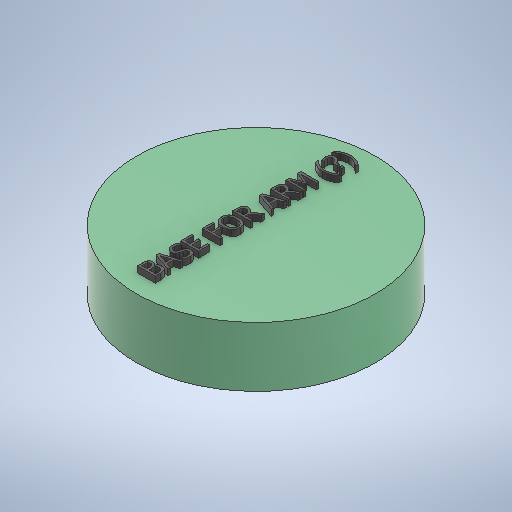
# Autodesk Inventor part: Base Mockup
Saved by Autodesk Inventor 2025.2 (Build 292293000, 293)
## iProperties
Created: 2025-01-24
Part Number: Base Mockup
Material: Generic
Document SubType Name: Modeling
Designer: Matt Tidd
Density: 1 g/cm^3
Appearance: Default
Author: Matt Tidd
Autodesk Inventor part; units mm, degrees
ref_plane "YZ Plane" through (0, 0, 0) normal (1, 0, 0) x (0, 1, 0)
ref_plane "XZ Plane" through (0, 0, 0) normal (0, 1, 0) x (-1, 0, 0)
ref_plane "XY Plane" through (0, 0, 0) normal (0, 0, 1) x (1, 0, 0)
sketch "Sketch1" plane through (0, 0, 0) normal (0, 1, 0) x (-1, 0, 0)
  circle A0 centre (0, 0) radius 50
  dimension "d0" = 100
  constraints: 1 centre point, 1 coincident
  measures "d0" diameter of A0
extrude "Extrusion1" add sketch "Sketch1" along normal blind 25
sketch "Sketch2" plane through (0, 25, 0) normal (0, 1, 0) x (1, 0, 0)
  line L0 (0, -50) -> (0, 50) construction
  circle A0 centre (0, 0) radius 50 projected
  spline S0 degree 2 poles (-2.3035, -37.0837) (-1.7443, -37.0837) (-0.8874, -37.5091) (-0.6078, -37.8616) knots 0 0 0 1 2 2 2
  spline S1 degree 2 poles (-0.6078, -37.8616) (-0.2796, -38.2871) (0, -39.2534) (0, -40.0192) knots 0 0 0 1 2 2 2
  line L1 (0, -40.0192) -> (0, -42.1708)
  line L2 (0, -42.1708) -> (-7.5, -42.1708)
  line L3 (-7.5, -42.1708) -> (-7.5, -40.1833)
  spline S2 degree 2 poles (-7.5, -40.1833) (-7.5, -39.3811) (-7.3967, -38.5788) (-7.1961, -38.2141) knots 0 0 0 1 2 2 2
  spline S3 degree 2 poles (-7.1961, -38.2141) (-6.9834, -37.8069) (-6.2844, -37.4362) (-5.8104, -37.4362) knots 0 0 0 1 2 2 2
  spline S4 degree 2 poles (-5.8104, -37.4362) (-5.2816, -37.4362) (-4.4429, -37.9953) (-4.2058, -38.4876) knots 0 0 0 1 2 2 2
  line L4 (-4.2058, -38.4876) -> (-4.1694, -38.4876)
  spline S5 degree 2 poles (-4.1694, -38.4876) (-3.987, -37.8191) (-3.0207, -37.0837) (-2.3035, -37.0837) knots 0 0 0 1 2 2 2
  spline S6 degree 2 poles (-2.2609, -38.123) (-2.6864, -38.123) (-3.2334, -38.3661) (-3.4279, -38.7308) knots 0 0 0 1 2 2 2
  spline S7 degree 2 poles (-3.4279, -38.7308) (-3.5494, -38.9678) (-3.6224, -39.5269) (-3.6224, -40.0436) knots 0 0 0 1 2 2 2
  line L5 (-3.6224, -40.0436) -> (-3.6224, -41.174)
  line L6 (-3.6224, -41.174) -> (-0.8509, -41.174)
  line L7 (-0.8509, -41.174) -> (-0.8509, -40.3657)
  spline S8 degree 2 poles (-0.8509, -40.3657) (-0.8509, -39.7093) (-0.9724, -38.9556) (-1.1669, -38.6639) knots 0 0 0 1 2 2 2
  spline S9 degree 2 poles (-1.1669, -38.6639) (-1.3675, -38.3843) (-1.8659, -38.123) (-2.2609, -38.123) knots 0 0 0 1 2 2 2
  spline S10 degree 2 poles (-5.6706, -38.4755) (-5.938, -38.4755) (-6.3391, -38.6578) (-6.4546, -38.8584) knots 0 0 0 1 2 2 2
  spline S11 degree 2 poles (-6.4546, -38.8584) (-6.5883, -39.1015) (-6.6491, -39.691) (-6.6491, -40.2198) knots 0 0 0 1 2 2 2
  line L8 (-6.6491, -40.2198) -> (-6.6491, -41.174)
  line L9 (-6.6491, -41.174) -> (-4.455, -41.174)
  line L10 (-4.455, -41.174) -> (-4.455, -40.0436)
  spline S12 degree 2 poles (-4.455, -40.0436) (-4.455, -39.5756) (-4.5523, -39.1319) (-4.7042, -38.8949) knots 0 0 0 1 2 2 2
  spline S13 degree 2 poles (-4.7042, -38.8949) (-4.8501, -38.6639) (-5.3181, -38.4755) (-5.6706, -38.4755) knots 0 0 0 1 2 2 2
  line L11 (0, -36.9013) -> (-7.5, -34.373)
  line L12 (-7.5, -34.373) -> (-7.5, -33.1453)
  line L13 (-7.5, -33.1453) -> (0, -30.6169)
  line L14 (0, -30.6169) -> (0, -31.6684)
  line L15 (0, -31.6684) -> (-2.0968, -32.3491)
  line L16 (-2.0968, -32.3491) -> (-2.0968, -35.2117)
  line L17 (-2.0968, -35.2117) -> (0, -35.8924)
  line L18 (0, -35.8924) -> (0, -36.9013)
  line L19 (-2.9477, -32.6226) -> (-6.4789, -33.7834)
  line L20 (-6.4789, -33.7834) -> (-2.9477, -34.9382)
  line L21 (-2.9477, -34.9382) -> (-2.9477, -32.6226)
  spline S14 degree 2 poles (0.1337, -27.7178) (0.1337, -28.5322) (-0.2066, -29.6748) (-0.4498, -30.1793) knots 0 0 0 1 2 2 2
  line L22 (-0.4498, -30.1793) -> (-1.7018, -30.1793)
  line L23 (-1.7018, -30.1793) -> (-1.7018, -30.1064)
  spline S15 degree 2 poles (-1.7018, -30.1064) (-1.2399, -29.6141) (-0.7293, -28.3681) (-0.7293, -27.7907) knots 0 0 0 1 2 2 2
  spline S16 degree 2 poles (-0.7293, -27.7907) (-0.7293, -26.9641) (-1.4161, -26.1193) (-1.9814, -26.1193) knots 0 0 0 1 2 2 2
  spline S17 degree 2 poles (-1.9814, -26.1193) (-2.4311, -26.1193) (-2.9903, -26.563) (-3.1301, -27.0432) knots 0 0 0 1 2 2 2
  spline S18 degree 2 poles (-3.1301, -27.0432) (-3.2273, -27.3896) (-3.361, -27.967) (-3.4704, -28.3985) knots 0 0 0 1 2 2 2
  spline S19 degree 2 poles (-3.4704, -28.3985) (-3.5737, -28.7875) (-3.8837, -29.4013) (-4.1329, -29.6384) knots 0 0 0 1 2 2 2
  spline S20 degree 2 poles (-4.1329, -29.6384) (-4.3821, -29.8693) (-5.0506, -30.1246) (-5.4882, -30.1246) knots 0 0 0 1 2 2 2
  spline S21 degree 2 poles (-5.4882, -30.1246) (-6.3999, -30.1246) (-7.6337, -28.7024) (-7.6337, -27.6023) knots 0 0 0 1 2 2 2
  spline S22 degree 2 poles (-7.6337, -27.6023) (-7.6337, -26.9702) (-7.3845, -25.8519) (-7.1475, -25.3718) knots 0 0 0 1 2 2 2
  line L24 (-7.1475, -25.3718) -> (-5.9562, -25.3718)
  line L25 (-5.9562, -25.3718) -> (-5.9562, -25.4447)
  spline S23 degree 2 poles (-5.9562, -25.4447) (-6.2844, -25.8033) (-6.7707, -26.9216) (-6.7707, -27.5355) knots 0 0 0 1 2 2 2
  spline S24 degree 2 poles (-6.7707, -27.5355) (-6.7707, -28.2283) (-6.1203, -29.0853) (-5.5916, -29.0853) knots 0 0 0 1 2 2 2
  spline S25 degree 2 poles (-5.5916, -29.0853) (-5.1175, -29.0853) (-4.5523, -28.5808) (-4.4246, -28.1068) knots 0 0 0 1 2 2 2
  spline S26 degree 2 poles (-4.4246, -28.1068) (-4.3395, -27.7907) (-4.1207, -26.873) (-4.0296, -26.5691) knots 0 0 0 1 2 2 2
  spline S27 degree 2 poles (-4.0296, -26.5691) (-3.7925, -25.7972) (-2.8383, -25.08) (-2.1394, -25.08) knots 0 0 0 1 2 2 2
  spline S28 degree 2 poles (-2.1394, -25.08) (-1.6957, -25.08) (-0.8448, -25.4386) (-0.547, -25.7607) knots 0 0 0 1 2 2 2
  spline S29 degree 2 poles (-0.547, -25.7607) (-0.2188, -26.1193) (0.1337, -27.031) (0.1337, -27.7178) knots 0 0 0 1 2 2 2
  line L26 (0, -24.065) -> (-7.5, -24.065)
  line L27 (-7.5, -24.065) -> (-7.5, -19.373)
  line L28 (-7.5, -19.373) -> (-6.6126, -19.373)
  line L29 (-6.6126, -19.373) -> (-6.6126, -23.0683)
  line L30 (-6.6126, -23.0683) -> (-4.5583, -23.0683)
  line L31 (-4.5583, -23.0683) -> (-4.5583, -19.6222)
  line L32 (-4.5583, -19.6222) -> (-3.671, -19.6222)
  line L33 (-3.671, -19.6222) -> (-3.671, -23.0683)
  line L34 (-3.671, -23.0683) -> (-0.8874, -23.0683)
  line L35 (-0.8874, -23.0683) -> (-0.8874, -19.373)
  line L36 (-0.8874, -19.373) -> (0, -19.373)
  line L37 (0, -19.373) -> (0, -24.065)
  line L38 (-6.6126, -10.5723) -> (-6.6126, -14.061)
  line L39 (-6.6126, -14.061) -> (-4.4976, -14.061)
  line L40 (-4.4976, -14.061) -> (-4.4976, -10.7182)
  line L41 (-4.4976, -10.7182) -> (-3.6102, -10.7182)
  line L42 (-3.6102, -10.7182) -> (-3.6102, -14.061)
  line L43 (-3.6102, -14.061) -> (0, -14.061)
  line L44 (0, -14.061) -> (0, -15.0577)
  line L45 (0, -15.0577) -> (-7.5, -15.0577)
  line L46 (-7.5, -15.0577) -> (-7.5, -10.5723)
  line L47 (-7.5, -10.5723) -> (-6.6126, -10.5723)
  spline S30 degree 2 poles (-6.643, -4.373) (-6.1447, -3.9475) (-4.686, -3.4735) (-3.75, -3.4735) knots 0 0 0 1 2 2 2
  spline S31 degree 2 poles (-3.75, -3.4735) (-2.8383, -3.4735) (-1.3614, -3.9354) (-0.863, -4.373) knots 0 0 0 1 2 2 2
  spline S32 degree 2 poles (-0.863, -4.373) (-0.3404, -4.8349) (0.158, -6.0565) (0.158, -6.7919) knots 0 0 0 1 2 2 2
  spline S33 degree 2 poles (0.158, -6.7919) (0.158, -7.5517) (-0.3586, -8.7672) (-0.863, -9.2109) knots 0 0 0 1 2 2 2
  spline S34 degree 2 poles (-0.863, -9.2109) (-1.3614, -9.6424) (-2.8262, -10.1043) (-3.75, -10.1043) knots 0 0 0 1 2 2 2
  spline S35 degree 2 poles (-3.75, -10.1043) (-4.6921, -10.1043) (-6.1264, -9.6363) (-6.643, -9.2048) knots 0 0 0 1 2 2 2
  spline S36 degree 2 poles (-6.643, -9.2048) (-7.1414, -8.7672) (-7.658, -7.5456) (-7.658, -6.7919) knots 0 0 0 1 2 2 2
  spline S37 degree 2 poles (-7.658, -6.7919) (-7.658, -6.0261) (-7.1232, -4.7984) (-6.643, -4.373) knots 0 0 0 1 2 2 2
  spline S38 degree 2 poles (-3.75, -4.5128) (-4.4915, -4.5128) (-5.6402, -4.8349) (-6.017, -5.1266) knots 0 0 0 1 2 2 2
  spline S39 degree 2 poles (-6.017, -5.1266) (-6.406, -5.4244) (-6.795, -6.2632) (-6.795, -6.7859) knots 0 0 0 1 2 2 2
  spline S40 degree 2 poles (-6.795, -6.7859) (-6.795, -7.3268) (-6.4182, -8.1412) (-6.017, -8.4512) knots 0 0 0 1 2 2 2
  spline S41 degree 2 poles (-6.017, -8.4512) (-5.6341, -8.749) (-4.4793, -9.065) (-3.75, -9.065) knots 0 0 0 1 2 2 2
  spline S42 degree 2 poles (-3.75, -9.065) (-2.2731, -9.065) (-0.705, -7.8252) (-0.705, -6.7859) knots 0 0 0 1 2 2 2
  spline S43 degree 2 poles (-0.705, -6.7859) (-0.705, -5.7466) (-2.2731, -4.5128) (-3.75, -4.5128) knots 0 0 0 1 2 2 2
  line L48 (0, 3.4248) -> (0, 2.1303)
  line L49 (0, 2.1303) -> (-2.9842, -0.2401)
  line L50 (-2.9842, -0.2401) -> (-2.9842, -1.3827)
  line L51 (-2.9842, -1.3827) -> (0, -1.3827)
  line L52 (0, -1.3827) -> (0, -2.3795)
  line L53 (0, -2.3795) -> (-7.5, -2.3795)
  line L54 (-7.5, -2.3795) -> (-7.5, -0.4467)
  spline S44 degree 2 poles (-7.5, -0.4467) (-7.5, 0.1975) (-7.3602, 1.0667) (-7.1049, 1.4617) knots 0 0 0 1 2 2 2
  spline S45 degree 2 poles (-7.1049, 1.4617) (-6.8497, 1.8568) (-6.0535, 2.3126) (-5.4639, 2.3126) knots 0 0 0 1 2 2 2
  spline S46 degree 2 poles (-5.4639, 2.3126) (-4.6434, 2.3126) (-3.5312, 1.4739) (-3.2638, 0.7567) knots 0 0 0 1 2 2 2
  line L55 (-3.2638, 0.7567) -> (0, 3.4248)
  spline S47 degree 2 poles (-5.3849, 1.2733) (-5.7131, 1.2733) (-6.2176, 1.0423) (-6.3817, 0.7992) knots 0 0 0 1 2 2 2
  spline S48 degree 2 poles (-6.3817, 0.7992) (-6.5215, 0.5865) (-6.637, 0.0213) (-6.637, -0.392) knots 0 0 0 1 2 2 2
  line L56 (-6.637, -0.392) -> (-6.637, -1.3827)
  line L57 (-6.637, -1.3827) -> (-3.8169, -1.3827)
  line L58 (-3.8169, -1.3827) -> (-3.8169, -0.5075)
  spline S49 degree 2 poles (-3.8169, -0.5075) (-3.8169, -0.076) (-3.9688, 0.6108) (-4.2058, 0.8479) knots 0 0 0 1 2 2 2
  spline S50 degree 2 poles (-4.2058, 0.8479) (-4.4125, 1.0667) (-4.9959, 1.2733) (-5.3849, 1.2733) knots 0 0 0 1 2 2 2
  line L59 (0, 6.4333) -> (-7.5, 8.9617)
  line L60 (-7.5, 8.9617) -> (-7.5, 10.1894)
  line L61 (-7.5, 10.1894) -> (0, 12.7178)
  line L62 (0, 12.7178) -> (0, 11.6663)
  line L63 (0, 11.6663) -> (-2.0968, 10.9856)
  line L64 (-2.0968, 10.9856) -> (-2.0968, 8.123)
  line L65 (-2.0968, 8.123) -> (0, 7.4423)
  line L66 (0, 7.4423) -> (0, 6.4333)
  line L67 (-2.9477, 10.7121) -> (-6.4789, 9.5513)
  line L68 (-6.4789, 9.5513) -> (-2.9477, 8.3965)
  line L69 (-2.9477, 8.3965) -> (-2.9477, 10.7121)
  line L70 (0, 19.3304) -> (0, 18.0359)
  line L71 (0, 18.0359) -> (-2.9842, 15.6655)
  line L72 (-2.9842, 15.6655) -> (-2.9842, 14.5229)
  line L73 (-2.9842, 14.5229) -> (0, 14.5229)
  line L74 (0, 14.5229) -> (0, 13.5261)
  line L75 (0, 13.5261) -> (-7.5, 13.5261)
  line L76 (-7.5, 13.5261) -> (-7.5, 15.4589)
  spline S51 degree 2 poles (-7.5, 15.4589) (-7.5, 16.1031) (-7.3602, 16.9722) (-7.1049, 17.3673) knots 0 0 0 1 2 2 2
  spline S52 degree 2 poles (-7.1049, 17.3673) (-6.8497, 17.7624) (-6.0535, 18.2182) (-5.4639, 18.2182) knots 0 0 0 1 2 2 2
  spline S53 degree 2 poles (-5.4639, 18.2182) (-4.6434, 18.2182) (-3.5312, 17.3795) (-3.2638, 16.6623) knots 0 0 0 1 2 2 2
  line L77 (-3.2638, 16.6623) -> (0, 19.3304)
  spline S54 degree 2 poles (-5.3849, 17.1789) (-5.7131, 17.1789) (-6.2176, 16.9479) (-6.3817, 16.7048) knots 0 0 0 1 2 2 2
  spline S55 degree 2 poles (-6.3817, 16.7048) (-6.5215, 16.4921) (-6.637, 15.9269) (-6.637, 15.5136) knots 0 0 0 1 2 2 2
  line L78 (-6.637, 15.5136) -> (-6.637, 14.5229)
  line L79 (-6.637, 14.5229) -> (-3.8169, 14.5229)
  line L80 (-3.8169, 14.5229) -> (-3.8169, 15.3981)
  spline S56 degree 2 poles (-3.8169, 15.3981) (-3.8169, 15.8296) (-3.9688, 16.5164) (-4.2058, 16.7534) knots 0 0 0 1 2 2 2
  spline S57 degree 2 poles (-4.2058, 16.7534) (-4.4125, 16.9722) (-4.9959, 17.1789) (-5.3849, 17.1789) knots 0 0 0 1 2 2 2
  line L81 (0, 26.3564) -> (0, 25.3596)
  line L82 (0, 25.3596) -> (-6.4607, 25.3596)
  line L83 (-6.4607, 25.3596) -> (-2.0665, 23.4026)
  line L84 (-2.0665, 23.4026) -> (-2.0665, 22.7948)
  line L85 (-2.0665, 22.7948) -> (-6.4607, 20.856)
  line L86 (-6.4607, 20.856) -> (0, 20.856)
  line L87 (0, 20.856) -> (0, 19.9261)
  line L88 (0, 19.9261) -> (-7.5, 19.9261)
  line L89 (-7.5, 19.9261) -> (-7.5, 21.2875)
  line L90 (-7.5, 21.2875) -> (-3.3246, 23.1594)
  line L91 (-3.3246, 23.1594) -> (-7.5, 24.9706)
  line L92 (-7.5, 24.9706) -> (-7.5, 26.3564)
  line L93 (-7.5, 26.3564) -> (0, 26.3564)
  line L94 (2.0725, 33.9111) -> (2.0725, 32.7563)
  spline S58 degree 2 poles (2.0725, 32.7563) (1.0332, 31.8811) (-1.2946, 30.8782) (-2.8809, 30.8782) knots 0 0 0 1 2 2 2
  spline S59 degree 2 poles (-2.8809, 30.8782) (-4.4307, 30.8782) (-6.795, 31.8689) (-7.8343, 32.7563) knots 0 0 0 1 2 2 2
  line L95 (-7.8343, 32.7563) -> (-7.8343, 33.9111)
  line L96 (-7.8343, 33.9111) -> (-7.7857, 33.9111)
  spline S60 degree 2 poles (-7.7857, 33.9111) (-7.4149, 33.5039) (-6.4546, 32.7624) (-5.8165, 32.4463) knots 0 0 0 1 2 2 2
  spline S61 degree 2 poles (-5.8165, 32.4463) (-5.1965, 32.1424) (-3.7075, 31.7656) (-2.8809, 31.7656) knots 0 0 0 1 2 2 2
  spline S62 degree 2 poles (-2.8809, 31.7656) (-2.0178, 31.7656) (-0.5895, 32.1303) (0.0547, 32.4463) knots 0 0 0 1 2 2 2
  spline S63 degree 2 poles (0.0547, 32.4463) (0.6746, 32.7502) (1.6775, 33.5221) (2.0239, 33.9111) knots 0 0 0 1 2 2 2
  line L97 (2.0239, 33.9111) -> (2.0725, 33.9111)
  spline S64 degree 2 poles (-5.7374, 38.8766) (-5.2451, 38.8766) (-4.4733, 38.5484) (-4.1815, 38.2749) knots 0 0 0 1 2 2 2
  spline S65 degree 2 poles (-4.1815, 38.2749) (-3.8898, 38.0075) (-3.3975, 37.3146) (-3.1665, 36.9317) knots 0 0 0 1 2 2 2
  line L98 (-3.1665, 36.9317) -> (-2.0178, 36.9317)
  line L99 (-2.0178, 36.9317) -> (-2.0178, 36.0322)
  line L100 (-2.0178, 36.0322) -> (-3.5555, 36.0322)
  spline S66 degree 2 poles (-3.5555, 36.0322) (-3.7257, 36.3118) (-4.1998, 37.0654) (-4.4064, 37.2782) knots 0 0 0 1 2 2 2
  spline S67 degree 2 poles (-4.4064, 37.2782) (-4.6677, 37.5456) (-5.2755, 37.8495) (-5.6645, 37.8495) knots 0 0 0 1 2 2 2
  spline S68 degree 2 poles (-5.6645, 37.8495) (-6.2297, 37.8495) (-6.7889, 37.1323) (-6.7889, 36.561) knots 0 0 0 1 2 2 2
  spline S69 degree 2 poles (-6.7889, 36.561) (-6.7889, 36.0565) (-6.4546, 35.1692) (-6.2723, 34.8896) knots 0 0 0 1 2 2 2
  line L101 (-6.2723, 34.8896) -> (-6.2723, 34.8349)
  line L102 (-6.2723, 34.8349) -> (-7.2994, 34.8349)
  spline S70 degree 2 poles (-7.2994, 34.8349) (-7.4331, 35.1692) (-7.6519, 36.1963) (-7.6519, 36.6582) knots 0 0 0 1 2 2 2
  spline S71 degree 2 poles (-7.6519, 36.6582) (-7.6519, 37.6915) (-6.6005, 38.8766) (-5.7374, 38.8766) knots 0 0 0 1 2 2 2
  line L103 (0, 37.0107) -> (0, 35.9897)
  line L104 (0, 35.9897) -> (-1.0636, 35.9897)
  line L105 (-1.0636, 35.9897) -> (-1.0636, 37.0107)
  line L106 (-1.0636, 37.0107) -> (0, 37.0107)
  spline S72 degree 2 poles (-2.8809, 42.5841) (-1.325, 42.5841) (1.0332, 41.5873) (2.0725, 40.706) knots 0 0 0 1 2 2 2
  line L107 (2.0725, 40.706) -> (2.0725, 39.5513)
  line L108 (2.0725, 39.5513) -> (2.0239, 39.5513)
  spline S73 degree 2 poles (2.0239, 39.5513) (1.6775, 39.9402) (0.6625, 40.7243) (0.0547, 41.016) knots 0 0 0 1 2 2 2
  spline S74 degree 2 poles (0.0547, 41.016) (-0.5956, 41.3321) (-2.0421, 41.6967) (-2.8809, 41.6967) knots 0 0 0 1 2 2 2
  spline S75 degree 2 poles (-2.8809, 41.6967) (-3.7135, 41.6967) (-5.1904, 41.326) (-5.8165, 41.016) knots 0 0 0 1 2 2 2
  spline S76 degree 2 poles (-5.8165, 41.016) (-6.4425, 40.7121) (-7.4392, 39.9342) (-7.7857, 39.5513) knots 0 0 0 1 2 2 2
  line L109 (-7.7857, 39.5513) -> (-7.8343, 39.5513)
  line L110 (-7.8343, 39.5513) -> (-7.8343, 40.706)
  spline S77 degree 2 poles (-7.8343, 40.706) (-6.795, 41.5812) (-4.4489, 42.5841) (-2.8809, 42.5841) knots 0 0 0 1 2 2 2
  constraints: 2 end point, 2 vertical, 1 midpoint, 1 point on circle
extrude "Extrusion2" add sketch "Sketch2" along normal blind 2.5 contours S0 S1 L1 L2 L3 S2 S3 S4 L4 S5 | L11 L12 L13 L14 L15 L16 L17 L18 | S14 L22 L23 S15 S16 S17 S18 S19 S20 S21 S22 L24 L25 S23 S24 S25 S26 S27 S28 S29 | L26 L27 L28 L29 L30 L31 L32 L33 L34 L35 L36 L37 | L38 L39 L40 L41 L42 L43 L44 L45 L46 L47 | S30 S31 S32 S33 S34 S35 S36 S37 | L48 L49 L50 L51 L52 L53 L54 S44 S45 S46 L55 | L59 L60 L61 L62 L63 L64 L65 L66 | L70 L71 L72 L73 L74 L75 L76 S51 S52 S53 L77 | L81 L82 L83 L84 L85 L86 L87 L88 L89 L90 L91 L92 L93 | L94 S58 S59 L95 L96 S60 S61 S62 S63 L97 | S64 S65 L98 L99 L100 S66 S67 S68 S69 L101 L102 S70 S71 | L103 L104 L105 L106 | S72 L107 L108 S73 S74 S75 S76 L109 L110 S77
body "Solid1"
